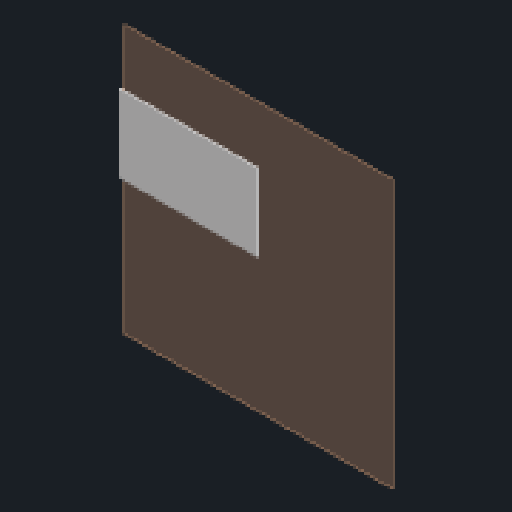
# Autodesk Inventor part: Antenna
Saved by Autodesk Inventor 2026.2 (Build 302298000, 298)
## iProperties
Created: 2026-05-11
Part Number: Antenna
Material: Polystyrene
Document SubType Name: Modeling
Designer: Malthe Sennels
Density: 1.021 g/cm^3
Appearance: Smooth - White
Author: Malthe Sennels
Autodesk Inventor part; units mm, degrees
ref_plane "YZ Plane" through (0, 0, 0) normal (1, 0, 0) x (0, 1, 0)
ref_plane "XZ Plane" through (0, 0, 0) normal (0, 1, 0) x (-1, 0, 0)
ref_plane "XY Plane" through (0, 0, 0) normal (0, 0, 1) x (1, 0, 0)
ref_plane "Work Plane1" through (25.4381, 4.2054, 4.72) normal (0, 0, 1) x (0.7071, 0.7071, 0)
sketch "Sketch1" plane through (25.4381, 4.2054, 4.72) normal (0, 0, 1) x (0.7071, 0.7071, 0)
  line L0 (-20.9611, 15.0138) -> (-186.9611, 15.0138)
  line L1 (-186.9611, 15.0138) -> (-186.9611, 95.0138)
  line L2 (-186.9611, 95.0138) -> (-20.9611, 95.0138)
  line L3 (-20.9611, 95.0138) -> (-20.9611, 15.0138)
  dimension "d0" = 166
  dimension "d1" = 80
  constraints: 8 end point, 2 parallel, 1 horizontal, 1 perpendicular
  measures "d0" distance of L1.end L2.end
  measures "d1" distance of L0.end L1.end
extrude "Extrusion1" add sketch "Sketch1" along normal blind 1.6
sketch "Sketch2" plane through (25.4381, 4.2054, 6.32) normal (0, 0, 1) x (0.7071, 0.7071, 0)
  point P0 (-20.9611, 15.0138)
sketch "Sketch3" plane through (25.4381, 4.2054, 6.32) normal (0, 0, 1) x (0.7071, -0.7071, 0)
  circle A0 centre (-103.5277, -22.9611) radius 1.6 projected
  circle A1 centre (-89.0425, -28.9611) radius 1.6 projected
  circle A2 centre (-20.9851, -28.9611) radius 1.6 projected
  point P0 (-15.0138, -20.9611)
ref_plane "Work Plane2" through (-28.2843, 28.2843, 4.72) normal (0.7071, -0.7071, 0) x (0, 0, 1)
extrude "Extrusion2" cut sketch "Sketch3" against normal blind 10 contours A1 | A2
sketch "Sketch4" plane through (25.4381, 4.2054, 6.32) normal (0, 0, 1) x (0.7071, -0.7071, 0)
  line L0 (-15.0138, -20.9611) -> (-95.0138, -20.9611) projected
  line L1 (-55.0138, -20.9611) -> (-55.0138, -186.9611) construction
  line L2 (-95.0138, -186.9611) -> (-15.0138, -186.9611) projected
  line L3 (-57.5138, -51.8936) -> (-52.5138, -51.8936)
  line L4 (-52.5138, -51.8936) -> (-52.5138, -20.9611)
  line L5 (-52.5138, -20.9611) -> (-57.5138, -20.9611)
  line L6 (-57.5138, -20.9611) -> (-57.5138, -51.8936)
  line L7 (-57.5138, -51.8936) -> (-52.5138, -20.9611) construction
  line L8 (-52.5138, -51.8936) -> (-57.5138, -20.9611) construction
  line L9 (-52.5138, -51.8936) -> (-77.9131, -51.8936)
  line L10 (-77.9131, -51.8936) -> (-77.9131, -46.8936)
  line L11 (-77.9131, -46.8936) -> (-52.5138, -46.8936)
  line L12 (-52.5138, -46.8936) -> (-52.5138, -51.8936)
  line L13 (-74.9089, -76.3936) -> (-35.1187, -76.3936)
  line L14 (-35.1187, -76.3936) -> (-35.1187, -72.3936)
  line L15 (-35.1187, -72.3936) -> (-74.9089, -72.3936)
  line L16 (-74.9089, -72.3936) -> (-74.9089, -76.3936)
  line L17 (-74.9089, -76.3936) -> (-35.1187, -72.3936) construction
  line L18 (-35.1187, -76.3936) -> (-74.9089, -72.3936) construction
  line L19 (-35.1187, -97.3936) -> (-74.9089, -97.3936)
  line L20 (-74.9089, -101.3936) -> (-35.1187, -97.3936) construction
  line L21 (-74.9089, -101.3936) -> (-35.1187, -101.3936)
  line L22 (-35.1187, -101.3936) -> (-74.9089, -97.3936) construction
  line L23 (-74.9089, -97.3936) -> (-74.9089, -101.3936)
  line L24 (-35.1187, -101.3936) -> (-35.1187, -97.3936)
  line L25 (-35.1187, -122.3936) -> (-74.9089, -122.3936)
  line L26 (-74.9089, -126.3936) -> (-35.1187, -122.3936) construction
  line L27 (-74.9089, -126.3936) -> (-35.1187, -126.3936)
  line L28 (-35.1187, -126.3936) -> (-74.9089, -122.3936) construction
  line L29 (-74.9089, -122.3936) -> (-74.9089, -126.3936)
  line L30 (-35.1187, -126.3936) -> (-35.1187, -122.3936)
  line L31 (-35.1187, -147.3936) -> (-74.9089, -147.3936)
  line L32 (-74.9089, -151.3936) -> (-35.1187, -147.3936) construction
  line L33 (-74.9089, -151.3936) -> (-35.1187, -151.3936)
  line L34 (-35.1187, -151.3936) -> (-74.9089, -147.3936) construction
  line L35 (-74.9089, -147.3936) -> (-74.9089, -151.3936)
  line L36 (-35.1187, -151.3936) -> (-35.1187, -147.3936)
  line L37 (-35.1187, -172.3936) -> (-74.9089, -172.3936)
  line L38 (-74.9089, -176.3936) -> (-35.1187, -172.3936) construction
  line L39 (-74.9089, -176.3936) -> (-35.1187, -176.3936)
  line L40 (-35.1187, -176.3936) -> (-74.9089, -172.3936) construction
  line L41 (-74.9089, -172.3936) -> (-74.9089, -176.3936)
  line L42 (-35.1187, -176.3936) -> (-35.1187, -172.3936)
  point P0 (-55.0138, -36.4274)
  point P1 (-55.0138, -74.3936)
  point P2 (-52.5138, -49.3936)
  point P3 (-55.0138, -99.3936)
  point P4 (-55.0138, -124.3936)
  point P5 (-55.0138, -149.3936)
  point P6 (-55.0138, -174.3936)
  point P7 (-57.5138, -51.8936)
  point P8 (-57.5138, -20.9611)
  point P9 (-57.5138, -46.8936)
  dimension "d7" = 5
  dimension "d8" = 5
  dimension "d9" = 4
  dimension "d10" = 25
  dimension "d13" = 25
  constraints: 82 end point, 7 midpoint, 6 parallel, 3 horizontal, 3 perpendicular, 3 point on line, 1 vertical, 44 other
  measures "d7" distance between parallel lines of L6 L4
  measures "d8" distance between parallel lines of L9 L11
  measures "d9" distance of L13.end L14.end
  measures "d10" vertical distance of point (-52.514, -49.394) point (-55.014, -74.394)
  measures "d13" distance of L14.end L19.start
extrude "Extrusion3" add sketch "Sketch4" along normal blind 0.1
equation "\"d13\" = d10"
body "Solid1"
